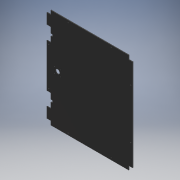
# Autodesk Inventor part: Internal Base Cladding
Saved by Autodesk Inventor 2017.3 (Build 213256000, 256)
## iProperties
Created: 2018-10-07
Part Number: Internal Base Cladding
Material: Aluminum 6061
Document SubType Name: Sheet Metal
Designer: Ax
Density: 2.7 g/cm^3
Appearance: Smooth - Black
Sheet Metal Rule: Default_mm
Author: Ax
Autodesk Inventor part; units mm, degrees
ref_plane "YZ Plane" through (0, 0, 0) normal (1, 0, 0) x (0, 1, 0)
ref_plane "XZ Plane" through (0, 0, 0) normal (0, 1, 0) x (-1, 0, 0)
ref_plane "XY Plane" through (0, 0, 0) normal (0, 0, 1) x (1, 0, 0)
sketch "Sketch1" plane through (0, 0, 0) normal (0, 1, 0) x (-1, 0, 0)
  line L0 (-220, 255) -> (220, 255)
  line L1 (220, 255) -> (220, -255)
  line L2 (220, -255) -> (-220, -255)
  line L3 (-220, -255) -> (-220, 255)
  line L4 (-220, 255) -> (220, -255) construction
  line L5 (220, 255) -> (-220, -255) construction
  line L6 (200, 255) -> (200, 235)
  line L7 (200, 235) -> (220, 235)
  line L8 (200, -255) -> (200, -235)
  line L9 (200, -235) -> (220, -235)
  line L10 (-200, 255) -> (-200, 235)
  line L11 (-200, 235) -> (-220, 235)
  line L12 (-200, -255) -> (-200, -235)
  line L13 (-200, -235) -> (-220, -235)
  point P0 (0, 0)
  dimension "d0" = 510
  dimension "d1" = 440
  dimension "d2" = 20
  constraints: 28 end point, 8 point on line, 7 equal length, 7 perpendicular, 2 horizontal, 2 midpoint, 2 parallel, 1 vertical
  measures "d0" distance of L0.end L1.end
  measures "d1" distance of L1.end L2.end
  measures "d2" distance of L8.end L8.start
extrude "Extrusion2" add sketch "Sketch1" along normal mid plane 3 contours L0 L6 L7 L1 L9 L8 L2 L12 L13 L3 L11 L10
sketch "Sketch2" plane through (0, -1.5, 0) normal (0, -1, 0) x (1, 0, 0)
  line L0 (210, -245) -> (-210, -245) construction
  line L1 (-210, -245) -> (-210, 245) construction
  line L2 (-210, 245) -> (210, 245) construction
  line L3 (210, 245) -> (210, -245) construction
  line L4 (210, -245) -> (-210, 245) construction
  line L5 (-210, -245) -> (210, 245) construction
  line L6 (-220, 235) -> (-220, -235) construction
  line L7 (200, 255) -> (-200, 255) construction
  circle A0 centre (-210, 98) radius 2.1
  circle A1 centre (-210, -98) radius 2.1
  circle A2 centre (-110, -245) radius 2.1
  circle A3 centre (110, -245) radius 2.1
  circle A4 centre (210, -127.5) radius 2.1
  circle A5 centre (210, 127.5) radius 2.1
  circle A6 centre (110, 245) radius 2.1
  circle A7 centre (-110, 245) radius 2.1
  line L8 (-220, 0) -> (220, 0) construction
  line L9 (-200, 255) -> (200, 255) construction
  line L10 (0, 255) -> (0, -257) construction
  point P0 (0, 0)
  point P1 (0, 0)
  point P2 (0, 0)
  dimension "d7" = 10
  dimension "d8" = 10
  dimension "d9" = 117.5
  dimension "d10" = 100
  dimension "d11" = 4.2
  dimension "d27" = 147
  constraints: 16 end point, 9 point on line, 8 centre point, 7 equal radius, 7 midpoint, 3 symmetric about line, 2 horizontal, 2 parallel, 2 perpendicular
  measures "d7" distance between parallel lines of L1 L6
  measures "d8" distance between parallel lines of L2 L7
  measures "d9" distance of L2.end A5.centre
  measures "d10" distance of L2.end A6.centre
  measures "d11" diameter of A7
  measures "d27" distance of A1.centre L0.end
extrude "Extrusion3" cut sketch "Sketch2" against normal through all
sketch "Sketch3" plane through (0, -1.5, 0) normal (0, -1, 0) x (1, 0, 0)
  line L0 (-180, -15.5) -> (-149, -15.5) construction
  line L1 (-149, -15.5) -> (-149, 15.5) construction
  line L2 (-149, 15.5) -> (-180, 15.5) construction
  line L3 (-180, 15.5) -> (-180, -15.5) construction
  line L4 (-180, -15.5) -> (-149, 15.5) construction
  line L5 (-149, -15.5) -> (-180, 15.5) construction
  line L6 (-220, 235) -> (-220, -235) projected
  line L7 (0, 0) -> (-220, 0) construction
  circle A0 centre (-164.5, 0) radius 11
  circle A1 centre (-180, 15.5) radius 1.7
  circle A2 centre (-149, 15.5) radius 1.7
  circle A3 centre (-149, -15.5) radius 1.7
  circle A4 centre (-180, -15.5) radius 1.7
  point P0 (-164.5, 0)
  dimension "d14" = 40
  dimension "d15" = 22
  dimension "d16" = 31
  dimension "d17" = 3.4
  constraints: 14 end point, 5 centre point, 5 coincident, 4 midpoint, 3 equal radius, 2 parallel, 2 perpendicular, 1 horizontal, 1 point on line
  measures "d14" distance between parallel lines of L3 L6
  measures "d15" diameter of A0
  measures "d16" distance of L0.end L1.end
  measures "d17" diameter of A2
extrude "Extrusion4" cut sketch "Sketch3" against normal through all
sketch "Sketch4" plane through (0, -1.5, 0) normal (0, -1, 0) x (1, 0, 0)
  line L0 (-220, 111.25) -> (-200, 111.25)
  line L1 (-200, 111.25) -> (-200, 181.75)
  line L2 (-200, 181.75) -> (-220, 181.75)
  line L3 (-220, 181.75) -> (-220, 111.25)
  line L4 (-200, 235) -> (-220, 235) projected
  line L5 (-220, 235) -> (-220, -235) projected
  line L6 (-220, 146.5) -> (-191, 146.5) construction
  line L7 (-200, 140.25) -> (-191.5, 140.25)
  line L8 (-191.5, 140.25) -> (-191.5, 152.75)
  line L9 (-191.5, 152.75) -> (-200, 152.75)
  line L10 (-200, 152.75) -> (-200, 140.25)
  point P0 (0, 0)
  dimension "d21" = 70.5
  dimension "d22" = 12.5
  dimension "d23" = 8.5
  dimension "d28" = 20
  dimension "d29" = 88.5
  constraints: 18 end point, 4 parallel, 3 horizontal, 3 point on line, 2 perpendicular, 2 symmetric about line
  measures "d21" distance of L0.end L1.end
  measures "d22" distance of L7.end L8.end
  measures "d23" distance of L8.end L9.end
  measures "d28" distance of L1.end L2.end
  measures "d29" distance of L4.end L6.start
extrude "Extrusion5" cut sketch "Sketch4" against normal through all
mirror "Mirror1" about plane through (0, 0, 0) normal (0, 0, 1) of "Extrusion5"
fillet "Fillet1" radius 1 12 edges at (-200, 0, -111.25) (-191.5, 0, -140.25) (-191.5, 0, -152.75) (-200, 0, -181.75) (-200, 0, -152.75) (-200, 0, -140.25) (-200, 0, 152.75) (-200, 0, 140.25) (-191.5, 0, 152.75) (-200, 0, 181.75) (-191.5, 0, 140.25) (-200, 0, 111.25)
equation "\"BendRadius\" = Thickness"
equation "\"BendReliefWidth\" = Thickness"
equation "\"BendReliefDepth\" = 0.5 * Thickness"
equation "\"CornerReliefSize\" = 4 * Thickness"
equation "\"MinimumRemnant\" = 2 * Thickness"
equation "\"TransitionRadius\" = BendRadius"
equation "\"JacobiRadiusSize\" = BendRadius"
equation "\"GapSize\" = Thickness"
equation "\"Thickness\" = 3"
body "Solid2"
